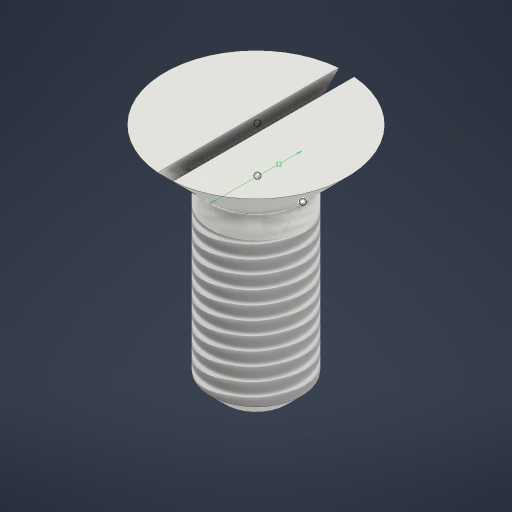
# Autodesk Inventor part: csk.screw
Saved by Autodesk Inventor 2023 (Build 270158000, 158)
## iProperties
Created: 2023-03-09
Part Number: csk.screw
Material: Steel, High Strength, Low Alloy
Document SubType Name: Modeling
Designer: kamraj
Density: 7.85 g/cm^3
Appearance: Steel
Author: kamraj
Autodesk Inventor part; units mm, degrees
ref_plane "YZ Plane" through (0, 0, 0) normal (1, 0, 0) x (0, 1, 0)
ref_plane "XZ Plane" through (0, 0, 0) normal (0, 1, 0) x (-1, 0, 0)
ref_plane "XY Plane" through (0, 0, 0) normal (0, 0, 1) x (1, 0, 0)
sketch "Sketch1" plane through (0, 0, 0) normal (0, 1, 0) x (-1, 0, 0)
  circle A0 centre (0, 0) radius 6
  dimension "d0" = 12
  constraints: 1 centre point, 1 coincident
  measures "d0" diameter of A0
extrude "Extrusion1" add sketch "Sketch1" along normal blind 6 draft 45
extrude "Extrusion2" add sketch "Sketch1" against normal blind 24
chamfer "Chamfer1" distance 2 angle 45 1 edges at (6, -24, 0)
thread "Thread1" size "M12x1.75" class "6g" standard "ANSI Metric M Profile" length 155 offset 3
sketch "Sketch2" plane through (0, 6, 0) normal (0, 1, 0) x (1, 0, 0)
  line L0 (1, -12) -> (1, 12)
  line L1 (1, 12) -> (-1, 12)
  line L2 (-1, 12) -> (-1, -12)
  line L3 (-1, -12) -> (1, -12)
  line L4 (1, -12) -> (-1, 12) construction
  line L5 (1, 12) -> (-1, -12) construction
  point P0 (0, 0)
  dimension "d10" = 2
  constraints: 12 end point, 2 midpoint, 2 parallel, 1 perpendicular, 1 vertical
  measures "d10" distance of L1.end L0.end
extrude "Extrusion3" cut sketch "Sketch2" against normal blind 3
body "Solid1"
